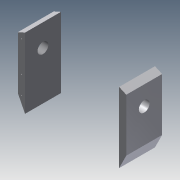
# Autodesk Inventor part: zadni_strana
Saved by Autodesk Inventor 2013 (Build 170138000, 138)
## iProperties
Created: 2012-08-22
Part Number: zadni_strana
Material: Generic
Document SubType Name: Modeling
Designer: idle-rug
Density: 1 g/cm^3
Author: idle-rug
Autodesk Inventor part; units mm, degrees
ref_plane "YZ Plane" through (0, 0, 0) normal (1, 0, 0) x (0, 1, 0)
ref_plane "XZ Plane" through (0, 0, 0) normal (0, 1, 0) x (-1, 0, 0)
ref_plane "XY Plane" through (0, 0, 0) normal (0, 0, 1) x (1, 0, 0)
sketch "Sketch1" plane through (0, 0, 0) normal (0, 1, 0) x (-1, 0, 0)
  line L0 (65.5, 36.75) -> (75.5, 36.75)
  line L1 (75.5, 36.75) -> (75.5, -36.75)
  line L2 (75.5, -36.75) -> (65.5, -36.75)
  line L3 (75.5, -36.75) -> (65.5, -56.75)
  line L4 (75.5, 36.75) -> (65.5, 41.1944)
  line L5 (-65.5, 36.75) -> (-75.5, 36.75)
  line L6 (-75.5, 36.75) -> (-75.5, -36.75)
  line L7 (-75.5, -36.75) -> (-65.5, -36.75)
  line L8 (-65.5, -56.75) -> (-75.5, -36.75)
  line L9 (-75.5, 36.75) -> (-65.5, 41.1944)
  line L10 (65.5, -56.75) -> (65.5, 41.1944)
  line L11 (-65.5, -56.75) -> (-65.5, 41.1944)
  dimension "d3" = 10
  dimension "d4" = 73.5
  dimension "d5" = 10
  dimension "d8" = 10
  dimension "d9" = 73.5
  constraints: 24 end point, 1 parallel, 1 perpendicular
  measures "d3" distance of L0.start L0.end
  measures "d4" distance of L0.end L1.end
  measures "d5" distance of L1.end L2.end
  measures "d8" distance of L5.start L5.end
  measures "d9" distance of L5.end L6.end
extrude "Extrusion1" add sketch "Sketch1" along normal blind 50
sketch "Sketch2" plane through (75.5, 0, 36.75) normal (1, 0, 0) x (0, 0, -1)
  circle A0 centre (26.5, 25) radius 7.5
  dimension "d16" = 15
  constraints: 1 centre point
  measures "d16" diameter of A0
hole "Hole1" at (75.5, 25, 10.25) direction (-1, 0, 0) diameter 15 depth 151
sketch "Sketch3" plane through (0, 0, 0) normal (0, -1, 0) x (1, 0, 0)
  line L0 (-65.5, -56.75) -> (-75.5, -36.75) projected
  line L1 (-65.5, 41.1944) -> (-65.5, -56.75) projected
  line L2 (-75.5, -36.75) -> (-75.5, 36.75) projected
  line L3 (-75.5, 36.75) -> (-75.5, 31.75)
  line L4 (-75.5, 31.75) -> (-70.5, 31.75)
  line L5 (-75.5, 36.75) -> (-75.5, -11.25)
  line L6 (-75.5, -11.25) -> (-70.5, -11.25)
  line L7 (-75.5, 36.75) -> (-75.5, -36.75)
  line L8 (-75.5, -36.75) -> (-70.5, -36.75)
  circle A0 centre (-70.5, 31.75) radius 3.4428
  circle A1 centre (-70.5, -11.25) radius 5.0721
  circle A2 centre (-70.5, -36.75) radius 4.4721
  point P0 (0, 0)
  dimension "d24" = 5
  dimension "d25" = 5
  dimension "d26" = 48
  dimension "d27" = 5
  dimension "d28" = 5
  constraints: 12 end point, 3 centre point, 3 coincident, 3 perpendicular, 2 point on line, 1 collinear, 1 tangent
  measures "d24" distance of L2.end L3.end
  measures "d25" distance of L3.end L4.end
  measures "d26" distance of L2.end L5.end
  measures "d27" distance of L5.end L6.end
  measures "d28" distance of L0.end L8.end
hole "Hole2" at (-70.5, 0, 31.75) at (-70.5, 0, -11.25) at (-70.5, 0, -36.75) direction (0, 1, 0) diameter 2 depth 50
body "Solid1"
